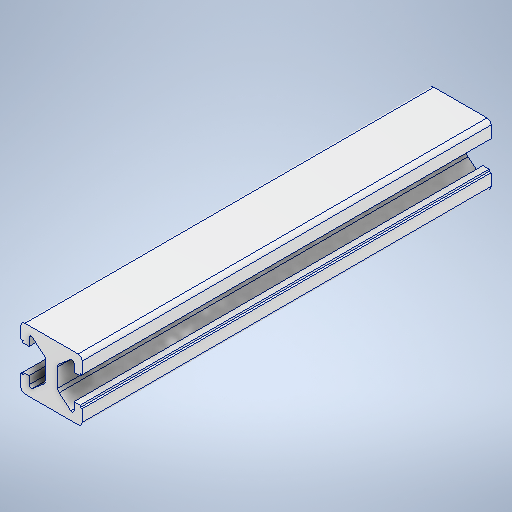
# Autodesk Inventor part: perfil_15x15_001
Saved by Autodesk Inventor 2025.2 (Build 292293000, 293)
## iProperties
Created: 2025-03-25
Part Number: perfil_15x15_001
Material: Alumínio 6061
Document SubType Name: Modeling
Designer: Carlos Dias
Density: 2.7 g/cm^3
Appearance: Alumínio - Plano
Author: Carlos Dias
Autodesk Inventor part; units mm, degrees
ref_plane "YZ Plane" through (0, 0, 0) normal (1, 0, 0) x (0, 1, 0)
ref_plane "XZ Plane" through (0, 0, 0) normal (0, 1, 0) x (-1, 0, 0)
ref_plane "XY Plane" through (0, 0, 0) normal (0, 0, 1) x (1, 0, 0)
sketch "Esboço1" plane through (0, 0, 0) normal (0, 0, 1) x (1, 0, 0)
  line L0 (-7.5, 7.5) -> (7.5, 7.5) construction
  line L1 (-7.5, 7.5) -> (-7.5, 3.1) construction
  line L2 (-7.5, 3.1) -> (-5.5, 3.1) construction
  line L3 (-5.5, 6.1) -> (-5.5, 3.1) construction
  line L4 (-5.5, 6.1) -> (-1.5, 2.7436) construction
  line L5 (-1.5, 2.7436) -> (-1.5, 0) construction
  line L6 (-1.5, 0) -> (0, 0)
  line L7 (0, 0) -> (0, 7.5)
  arc A0 (-6.5, 7.5) -> (-7.5, 6.5) centre (-6.5, 6.5) ccw
  arc A1 (-4.6786, 5.4108) -> (-5.5, 5.0277) centre (-5, 5.0277) ccw
  arc A2 (-1.5, 2.2773) -> (-1.8572, 3.0433) centre (-2.5, 2.2773) ccw
  line L8 (-7.5, 3.1) -> (-7, 3.1) construction
  line L9 (-7, 3.1) -> (-7, 3.6)
  line L10 (-7, 3.6) -> (-7.5, 3.6)
  line L11 (-7.5, 3.6) -> (-7.5, 3.1) construction
  line L12 (-7.5, 6.5) -> (-7.5, 3.6)
  line L13 (-7, 3.1) -> (-5.5, 3.1)
  line L14 (-5.5, 5.0277) -> (-5.5, 3.1)
  line L15 (-4.6786, 5.4108) -> (-1.8572, 3.0433)
  line L16 (-1.5, 0) -> (-1.5, 2.2773)
  line L17 (-6.5, 7.5) -> (0, 7.5)
  point P0 (-7.5, 5.3)
  dimension "d0" = 15
  dimension "d2" = 7.5
  dimension "d3" = 3.1
  dimension "d4" = 2
  dimension "d5" = 3
  dimension "d6" = 6
  dimension "d7" = 50
  dimension "d10" = 1
  dimension "d11" = 0.5
  dimension "d12" = 1
  dimension "d13" = 0.5
  constraints: 36 end point, 6 point on circle, 6 point on line, 6 tangent, 4 collinear, 4 horizontal, 4 vertical, 3 centre point, 3 perpendicular, 2 midpoint, 2 parallel, 1 vertical alignment
  measures "d0" distance of L0.start L0.end
  measures "d2" distance from line of L6.end L0
  measures "d3" vertical distance of L6.end L1.end
  measures "d4" distance of L1.end L2.end
  measures "d5" distance of L3.start L2.end
  measures "d6" horizontal distance of L1.end L4.end
  measures "d7" angle of L4 L3
  measures "d10" radius of A0
  measures "d11" radius of A1
  measures "d12" radius of A2
  measures "d13" distance of L9.end L10.end
extrude "Extrusão1" add sketch "Esboço1" along normal mid plane 100
mirror "Espelhar1" about plane through (0, 0, 0) normal (1, 0, 0) of "Extrusão1"
mirror "Espelhar2" about plane through (0, 0, 0) normal (0, 1, 0) of "Extrusão1", "Espelhar1"
